Autodesk Inventor part; units mm, degrees
(part 2 of 2)
  arc A502 (47.339, 28.73) -> (48.101, 28.73) centre (47.72, 28.73) ccw
  arc A503 (48.101, 28.73) -> (47.339, 28.73) centre (47.72, 28.73) ccw
  arc A504 (47.339, 28.73) -> (48.101, 28.73) centre (47.72, 28.73) ccw
  arc A505 (48.101, 28.73) -> (47.339, 28.73) centre (47.72, 28.73) ccw
  arc A506 (49.879, 28.73) -> (50.641, 28.73) centre (50.26, 28.73) ccw
  arc A507 (50.641, 28.73) -> (49.879, 28.73) centre (50.26, 28.73) ccw
  arc A508 (49.879, 28.73) -> (50.641, 28.73) centre (50.26, 28.73) ccw
  arc A509 (50.641, 28.73) -> (49.879, 28.73) centre (50.26, 28.73) ccw
  arc A510 (52.419, 28.73) -> (53.181, 28.73) centre (52.8, 28.73) ccw
  arc A511 (53.181, 28.73) -> (52.419, 28.73) centre (52.8, 28.73) ccw
  arc A512 (52.419, 28.73) -> (53.181, 28.73) centre (52.8, 28.73) ccw
  arc A513 (53.181, 28.73) -> (52.419, 28.73) centre (52.8, 28.73) ccw
  arc A514 (54.959, 28.73) -> (55.721, 28.73) centre (55.34, 28.73) ccw
  arc A515 (55.721, 28.73) -> (54.959, 28.73) centre (55.34, 28.73) ccw
  arc A516 (54.959, 28.73) -> (55.721, 28.73) centre (55.34, 28.73) ccw
  arc A517 (55.721, 28.73) -> (54.959, 28.73) centre (55.34, 28.73) ccw
  arc A518 (57.499, 28.73) -> (58.261, 28.73) centre (57.88, 28.73) ccw
  arc A519 (58.261, 28.73) -> (57.499, 28.73) centre (57.88, 28.73) ccw
  arc A520 (57.499, 28.73) -> (58.261, 28.73) centre (57.88, 28.73) ccw
  arc A521 (58.261, 28.73) -> (57.499, 28.73) centre (57.88, 28.73) ccw
  arc A522 (60.039, 28.73) -> (60.801, 28.73) centre (60.42, 28.73) ccw
  arc A523 (60.801, 28.73) -> (60.039, 28.73) centre (60.42, 28.73) ccw
  arc A524 (60.039, 28.73) -> (60.801, 28.73) centre (60.42, 28.73) ccw
  arc A525 (60.801, 28.73) -> (60.039, 28.73) centre (60.42, 28.73) ccw
  arc A526 (62.579, 28.73) -> (63.341, 28.73) centre (62.96, 28.73) ccw
  arc A527 (63.341, 28.73) -> (62.579, 28.73) centre (62.96, 28.73) ccw
  arc A528 (62.579, 28.73) -> (63.341, 28.73) centre (62.96, 28.73) ccw
  arc A529 (63.341, 28.73) -> (62.579, 28.73) centre (62.96, 28.73) ccw
  arc A530 (65.119, 28.73) -> (65.881, 28.73) centre (65.5, 28.73) ccw
  arc A531 (65.881, 28.73) -> (65.119, 28.73) centre (65.5, 28.73) ccw
  arc A532 (65.119, 28.73) -> (65.881, 28.73) centre (65.5, 28.73) ccw
  arc A533 (65.881, 28.73) -> (65.119, 28.73) centre (65.5, 28.73) ccw
  arc A534 (67.659, 28.73) -> (68.421, 28.73) centre (68.04, 28.73) ccw
  arc A535 (68.421, 28.73) -> (67.659, 28.73) centre (68.04, 28.73) ccw
  arc A536 (67.659, 28.73) -> (68.421, 28.73) centre (68.04, 28.73) ccw
  arc A537 (68.421, 28.73) -> (67.659, 28.73) centre (68.04, 28.73) ccw
  arc A538 (70.199, 28.73) -> (70.961, 28.73) centre (70.58, 28.73) ccw
  arc A539 (70.961, 28.73) -> (70.199, 28.73) centre (70.58, 28.73) ccw
  arc A540 (70.199, 28.73) -> (70.961, 28.73) centre (70.58, 28.73) ccw
  arc A541 (70.961, 28.73) -> (70.199, 28.73) centre (70.58, 28.73) ccw
  arc A542 (72.739, 28.73) -> (73.501, 28.73) centre (73.12, 28.73) ccw
  arc A543 (73.501, 28.73) -> (72.739, 28.73) centre (73.12, 28.73) ccw
  arc A544 (72.739, 28.73) -> (73.501, 28.73) centre (73.12, 28.73) ccw
  arc A545 (73.501, 28.73) -> (72.739, 28.73) centre (73.12, 28.73) ccw
  arc A546 (75.279, 28.73) -> (76.041, 28.73) centre (75.66, 28.73) ccw
  arc A547 (76.041, 28.73) -> (75.279, 28.73) centre (75.66, 28.73) ccw
  arc A548 (75.279, 28.73) -> (76.041, 28.73) centre (75.66, 28.73) ccw
  arc A549 (76.041, 28.73) -> (75.279, 28.73) centre (75.66, 28.73) ccw
  arc A550 (77.819, 28.73) -> (78.581, 28.73) centre (78.2, 28.73) ccw
  arc A551 (78.581, 28.73) -> (77.819, 28.73) centre (78.2, 28.73) ccw
  arc A552 (77.819, 28.73) -> (78.581, 28.73) centre (78.2, 28.73) ccw
  arc A553 (78.581, 28.73) -> (77.819, 28.73) centre (78.2, 28.73) ccw
  arc A554 (89.59, 30.6) -> (89.59, 29.7) centre (89.59, 30.15) ccw
  arc A555 (89.59, 29.7) -> (89.59, 30.6) centre (89.59, 30.15) ccw
  arc A556 (89.59, 30.6) -> (89.59, 29.7) centre (89.59, 30.15) ccw
  arc A557 (89.59, 29.7) -> (89.59, 30.6) centre (89.59, 30.15) ccw
  arc A558 (87.05, 30.6) -> (87.05, 29.7) centre (87.05, 30.15) ccw
  arc A559 (87.05, 29.7) -> (87.05, 30.6) centre (87.05, 30.15) ccw
  arc A560 (87.05, 30.6) -> (87.05, 29.7) centre (87.05, 30.15) ccw
  arc A561 (87.05, 29.7) -> (87.05, 30.6) centre (87.05, 30.15) ccw
  arc A562 (84.51, 30.6) -> (84.51, 29.7) centre (84.51, 30.15) ccw
  arc A563 (84.51, 29.7) -> (84.51, 30.6) centre (84.51, 30.15) ccw
  arc A564 (84.51, 30.6) -> (84.51, 29.7) centre (84.51, 30.15) ccw
  arc A565 (84.51, 29.7) -> (84.51, 30.6) centre (84.51, 30.15) ccw
  line L242 (44.7388, 33.8709) -> (94, 33.8709)
  line L243 (94, 33.8709) -> (94, 24.2027)
  line L244 (94, 24.2027) -> (44.7388, 24.2027)
  line L245 (44.7388, 24.2027) -> (44.7388, 33.8709)
  line L246 (28.3727, 38.1472) -> (43.5417, 38.1472)
  line L247 (43.5417, 38.1472) -> (43.5417, 25.8726)
  line L248 (43.5417, 25.8726) -> (28.3727, 25.8726)
  line L249 (28.3727, 25.8726) -> (28.3727, 38.1472)
  line L250 (74.0995, 167.7239) -> (74.3631, 167.7239)
  line L251 (74.3631, 167.7239) -> (74.3631, 160.0343)
  line L252 (56, 167.7239) -> (55.975, 167.7239)
  line L253 (55.975, 167.7239) -> (55.975, 162.0343)
  arc A566 (73.9995, 167.8228) -> (74.0995, 167.7239) centre (74.0995, 167.8239) ccw
  arc A567 (53.975, 160.0343) -> (55.975, 162.0343) centre (53.975, 162.0343) ccw
  point P0 (0, 0)
  point P1 (0, 0)
  dimension "d1" = 194.7239
  dimension "d26" = 2
  constraints: 984 point on circle, 568 centre point, 508 end point, 40 coincident, 40 concentric, 10 parallel, 6 horizontal, 6 perpendicular, 4 tangent
  measures "d1" distance between parallel lines of L0 L2
  measures "d26" radius of A567
extrude "押し出し1" add sketch "スケッチ2" along normal blind 5.5 contours L3 L2 L1 L0
sketch "スケッチ3" plane through (0, 0, 0) normal (0, 0, -1) x (-1, 0, 0)
  point P0 (0, 0)
sketch "スケッチ4" plane through (0, 0, 0) normal (0, 0, -1) x (-1, 0, 0)
  line L0 (-0.0414, 0.0414) -> (-0.0414, 194.7653) projected
  line L1 (-130.0414, 194.7653) -> (-130.0414, 0.0414) projected
  line L2 (-97.5532, 51.6566) -> (-32.5292, 51.6566)
  line L3 (-32.5292, 51.6566) -> (-32.5292, 0.3486)
  line L4 (-32.5292, 0.3486) -> (-97.5532, 0.3486)
  line L5 (-97.5532, 0.3486) -> (-97.5532, 51.6566)
  circle A0 centre (-36.3392, 47.5926) radius 1.6
  circle A1 centre (-43.9592, 4.4126) radius 1.6
  point P0 (0, 0)
  dimension "d5" = 130
  dimension "d17" = 3.2
  dimension "d18" = 3.81
  dimension "d19" = 4.064
  dimension "d20" = 3.2
  dimension "d22" = 11.43
  constraints: 8 end point, 2 centre point, 2 parallel, 1 horizontal, 1 perpendicular
  measures "d5" distance between parallel lines of L0 L1
  measures "d17" diameter of A0
  measures "d18" distance from line of L3 A0.centre
  measures "d19" distance from line of L2 A0.centre
  measures "d20" diameter of A1
  measures "d22" distance from line of L3 A1.centre
sketch "スケッチ5" plane through (0, 0, 0) normal (0, 0, -1) x (-1, 0, 0)
  point P0 (0, 0)
sketch "スケッチ6" plane through (0, 0, 0) normal (0, 0, -1) x (-1, 0, 0)
  point P0 (0, 0)
extrude "押し出し3" cut sketch "スケッチ4" against normal blind 5.5 contours A0 | A1
sketch "スケッチ7" plane through (0, 0, 5.5) normal (0, 0, 1) x (1, 0, 0)
  point P0 (0, 0)
sketch "スケッチ8" plane through (0, 0, 0) normal (0, 0, -1) x (-1, 0, 0)
  circle A0 centre (-96.7304, 150.7233) radius 1.6
  circle A1 centre (-84.0304, 163.4233) radius 1.6
  point P0 (0, 0)
  dimension "d36" = 3.2
  dimension "d37" = 3.2
  dimension "d38" = 12.7
  dimension "d39" = 12.7
  constraints: 2 centre point
  measures "d36" diameter of A0
  measures "d37" diameter of A1
  measures "d38" horizontal distance of A0.centre A1.centre
  measures "d39" horizontal distance of A1.centre A0.centre
extrude "押し出し4" cut sketch "スケッチ8" against normal blind 5.5
sketch "スケッチ9" plane through (0, 0, 5.5) normal (0, 0, 1) x (1, 0, 0)
  line L0 (39.514, 146.0723) -> (92.6312, 146.0723)
  line L1 (92.6312, 146.0723) -> (92.6312, 107.6919)
  line L2 (92.6312, 107.6919) -> (39.514, 107.6919)
  line L3 (39.514, 107.6919) -> (39.514, 146.0723)
  line L4 (39.514, 86.9632) -> (90.526, 86.9632)
  line L5 (90.526, 86.9632) -> (90.526, 49.2306)
  line L6 (90.526, 49.2306) -> (39.514, 49.2306)
  line L7 (39.514, 49.2306) -> (39.514, 86.9632)
  point P0 (0, 0)
  constraints: 16 end point, 4 parallel, 2 horizontal, 2 perpendicular, 1 point on line
extrude "押し出し5" add sketch "スケッチ9" against normal blind 5.5
sketch "スケッチ10" plane through (0, 0, 5.5) normal (0, 0, 1) x (1, 0, 0)
  circle A0 centre (95.5414, 52.4033) radius 1.6 projected
  circle A1 centre (95.5414, 82.4033) radius 1.6 projected
  circle A2 centre (34.5414, 142.4033) radius 1.6 projected
  circle A3 centre (34.5414, 112.4033) radius 1.6 projected
  circle A4 centre (72.9414, 142.4033) radius 1.6
  circle A5 centre (72.9414, 112.4033) radius 1.6
  circle A6 centre (57.1414, 82.4033) radius 1.6
  circle A7 centre (57.1414, 52.4033) radius 1.6
  line L0 (44.7388, 33.8709) -> (44.7388, 24.2027) projected
  line L1 (43.5417, 25.8726) -> (43.5417, 38.1472) projected
  line L2 (44.7388, 33.8709) -> (43.5417, 33.8709)
  line L3 (43.5417, 33.8709) -> (43.5417, 25.8726)
  line L4 (43.5417, 25.8726) -> (44.7388, 25.8726)
  line L5 (44.7388, 25.8726) -> (44.7388, 33.8709)
  point P0 (0, 0)
  constraints: 8 end point, 4 centre point, 2 parallel, 1 horizontal, 1 perpendicular
extrude "押し出し6" cut sketch "スケッチ10" against normal blind 5.5 contours A4 | A5 | A6 | A7 | L0 L4 L1 L2
